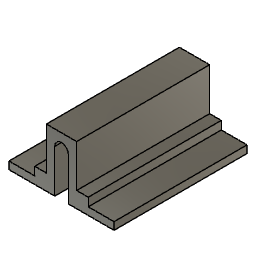
Stabilization tool v2 (Autodesk Fusion 360 design; units mm, degrees)
Autodesk Fusion 360 part; units mm, degrees
note: some values were not read from the file. Set by a fixed rule: which sketch regions a step uses.
sketch "Sketch1" plane through (0, 0, 0) normal (0, 1, 0) x (1, 0, 0)
  line L0 (-21.6, -69.1262) -> (2.8, -69.1262)
  line L1 (-21.6, -59.1262) -> (-21.6, -69.1262)
  line L2 (14.8, -18.1262) -> (28.8, -18.1262)
  line L3 (2.8, -69.1262) -> (14.8, -69.1262)
  line L4 (14.8, -59.1262) -> (14.8, -18.1262)
  line L5 (14.8, -69.1262) -> (14.8, -59.1262)
  line L6 (28.8, -18.1262) -> (28.8, -8.1262)
  line L7 (-66.6, -8.1262) -> (-35.6, -8.1262)
  line L8 (-66.6, 0.8738) -> (-66.6, -8.1262)
  line L9 (-21.6, -18.1262) -> (-35.6, -18.1262)
  line L10 (-35.6, -8.1262) -> (-66.6, -8.1262)
  line L11 (59.8, 0.8738) -> (59.8, -8.1262)
  line L12 (14.8, -18.1262) -> (14.8, -69.1262)
  line L13 (-35.6, -18.1262) -> (-35.6, -8.1262)
  line L14 (-21.6, -44.1262) -> (-21.6, -59.1262)
  line L15 (-21.6, -18.1262) -> (-21.6, -44.1262)
  line L16 (59.8, -8.1262) -> (28.8, -8.1262)
  line L17 (-35.6, -8.1262) -> (-35.6, -18.1262)
  line L18 (-35.6, -18.1262) -> (-21.6, -18.1262)
  line L19 (28.8, -8.1262) -> (28.8, -18.1262)
  line L20 (-21.6, -69.1262) -> (14.8, -69.1262)
  line L21 (-66.6, -8.1262) -> (-66.6, 0.8738)
  line L22 (-21.6, -69.1262) -> (-21.6, -18.1262)
  line L23 (28.8, -8.1262) -> (59.8, -8.1262)
  line L24 (59.8, -8.1262) -> (59.8, 0.8738)
  circle A0 centre (-3.4, -50.9262) radius 8.1
  line L25 (4.7, -50.9262) -> (-11.5, -50.9262) construction
  line L26 (-66.6, 0.8738) -> (59.8, 0.8738) construction
  line L27 (-11.5, -50.9262) -> (-11.5, 0.8738)
  line L28 (4.7, -50.9262) -> (4.7, 0.8738)
  line L29 (4.7, 0.8738) -> (59.8, 0.8738)
  line L30 (-11.5, 0.8738) -> (-66.6, 0.8738)
  point P0 (-3.2, -18.2523)
  dimension "d5" = 16.2
  constraint coincident L11.end L16.start
  constraint coincident L6.end L16.end
  constraint coincident L2.end L6.start
  constraint coincident L2.start L4.end
  constraint coincident L3.end L5.start
  constraint coincident L0.start L1.end
  constraint coincident L9.start L15.start
  constraint coincident L9.end L13.start
  constraint coincident L7.end L10.start
  constraint coincident L7.start L8.end
  constraint coincident L8.start L21.end
  constraint coincident L11.start L24.end
  constraint coincident A0 L25.start
  constraint coincident A0 L25.end
  constraint perpendicular L22 L25
  constraint perpendicular L21 L26
  constraint coincident L26 L27.end
  constraint tangent A0 L27
  constraint coincident L26 L28.end
  constraint tangent A0 L28
  constraint perpendicular L26 L28
  constraint perpendicular L11 L29
  constraint perpendicular L8 L30
  measures "d5" diameter of A0
extrude "Extrude1" add sketch "Sketch1" along normal blind 180 contours L0 L1 L2 L3 L4 L5 L6 L7 L8 L9 L10 L11 L12 L13 L14 L15 L16 L17 L18 L19 L20 L21 L22 L23 L24 A0 L27 L28 L29 L30
extrude "Extrude2" cut 1 faces at (-22.9, 180, 8.4595) along direction (0, -1, 0) blind 20
